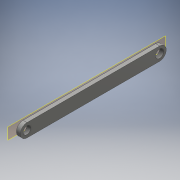
# Autodesk Inventor part: ServoLinkage_015
Saved by Autodesk Inventor 2016 (Build 200138000, 138)
## iProperties
Created: 2016-11-02
Part Number: ServoLinkage_015
Material: Generic
Document SubType Name: Modeling
Designer: mattc
Density: 1 g/cm^3
Appearance: Smooth - Medium Gray
Author: mattc
Autodesk Inventor part; units mm, degrees
ref_plane "YZ Plane" through (0, 0, 0) normal (1, 0, 0) x (0, 1, 0)
ref_plane "XZ Plane" through (0, 0, 0) normal (0, 1, 0) x (-1, 0, 0)
ref_plane "XY Plane" through (0, 0, 0) normal (0, 0, 1) x (1, 0, 0)
sketch "Sketch1" plane through (0, 0, 0) normal (1, 0, 0) x (0, 1, 0)
  circle A0 centre (0, 0) radius 2.875
  arc A1 (0, 5) -> (0, -5) centre (0, 0) ccw
  line L0 (0, 5) -> (100, 5)
  line L1 (100, -5) -> (0, -5)
  arc A2 (100, -5) -> (100, 5) centre (100, 0) ccw
  circle A3 centre (100, 0) radius 3.1
  dimension "d0" = 5.75
  dimension "d1" = 10
  dimension "d3" = 100
  dimension "d5" = 6.2
  dimension "d27" = 5
  constraints: 4 centre point, 4 end point, 4 point on circle, 3 coincident, 3 tangent, 1 horizontal, 1 parallel
  measures "d0" diameter of A0
  measures "d1" diameter of A1
  measures "d3" distance of L0.start L0.end
  measures "d5" diameter of A3
  measures "d27" radius of A2
extrude "Extrusion1" add sketch "Sketch1" along normal blind 3
ref_plane "Work Plane1" through (-2, 0, 0) normal (1, 0, 0) x (0, 0, -1)
equation "\"d27\" = 0.5 * d1"
body "Solid1"
